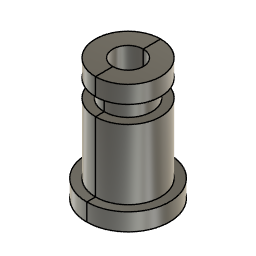
Befestigungsstift v1 (Autodesk Fusion 360 design; units mm, degrees)
Autodesk Fusion 360 part; units mm, degrees
sketch "Skizze1" plane through (0, 0, 0) normal (0, 1, 0) x (1, 0, 0)
  line L0 (0, -75) -> (0, 75)
  line L1 (3.75, -2.5) -> (-50.75, -2.5) construction
  line L2 (-50.75, -2.5) -> (-50.75, 2.5) construction
  line L3 (-50.75, 2.5) -> (49.25, 2.5) construction
  line L4 (49.25, 2.5) -> (49.25, -2.5) construction
  line L5 (1.75, 4.5) -> (4.75, 4.5)
  line L6 (4.75, 4.5) -> (4.75, 2.5)
  line L7 (3.75, 2.5) -> (3.75, -2.5)
  line L8 (3.75, -5.5) -> (2.75, -5.5)
  line L9 (2.75, -7.5) -> (3.75, -7.5)
  line L10 (3.75, -7.5) -> (3.75, -9.5)
  line L11 (3.75, -9.5) -> (1.75, -9.5)
  line L12 (1.75, -9.5) -> (1.75, 4.5)
  line L13 (49.25, -2.5) -> (3.75, -2.5) construction
  line L14 (3.75, -2.5) -> (3.75, -5.5)
  line L15 (3.75, 2.5) -> (4.75, 2.5)
  line L16 (2.75, -7.5) -> (2.75, -5.5)
  dimension "d1" = 100
  dimension "d2" = 5
  dimension "d3" = 2
  dimension "d4" = 2
  dimension "d5" = 3
  dimension "d6" = 2
  dimension "d7" = 1
  dimension "d8" = 3
  dimension "d9" = 5
  dimension "d10" = 2
  dimension "d11" = 7.5
  dimension "d12" = 1
  constraint vertical L0
  constraint horizontal L1
  constraint perpendicular L1 L2
  constraint parallel L1 L3
  constraint parallel L2 L4
  constraint parallel L3 L5
  constraint coincident L3 L6.end
  constraint perpendicular L5 L6
  constraint coincident L3 L7.start
  constraint perpendicular L1 L7
  constraint perpendicular L7 L8
  constraint perpendicular L9 L10
  constraint perpendicular L10 L11
  constraint perpendicular L5 L12
  constraint horizontal L13
  constraint perpendicular L1 L14
  constraint perpendicular L8 L16
  measures "d1" distance of L2.end L3.end
  measures "d2" distance of L1.end L2.end
  measures "d3" distance of L9.end L10.end
  measures "d4" distance of L8.end L9.start
  measures "d5" distance of L8.start L1.start
  measures "d6" distance of L5.end L6.end
  measures "d7" distance of L6.end L7.start
  measures "d8" distance of L5.start L5.end
  measures "d9" distance of L7.start L1.start
  measures "d10" distance of L10.end L11.end
  measures "d12" distance of L9.start L9.end
revolve "Drehen1" add sketch "Skizze1" angle 90 about axis through (0, 0, 75) along (0, 0, -1) second angle 90 makes body 1
mirror "Spiegeln1" about plane through (0, 0, 0) normal (1, 0, 0) of bodies 1 makes body 2
